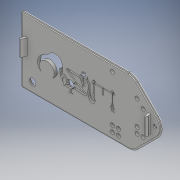
# Autodesk Inventor part: Arduino simple 4 channel ttl top
Saved by Autodesk Inventor 2017 (Build 210142000, 142)
## iProperties
Created: 2016-10-04
Part Number: Arduino simple 4 channel ttl top
Material: Generic
Document SubType Name: Modeling
Designer: andrew
Density: 1 g/cm^3
Appearance: Default
Author: andrew
Autodesk Inventor part; units mm, degrees
ref_plane "YZ Plane" through (0, 0, 0) normal (1, 0, 0) x (0, 1, 0)
ref_plane "XZ Plane" through (0, 0, 0) normal (0, 1, 0) x (-1, 0, 0)
ref_plane "XY Plane" through (0, 0, 0) normal (0, 0, 1) x (1, 0, 0)
sketch "Sketch1" plane through (0, 0, 0) normal (0, 1, 0) x (-1, 0, 0)
  line L0 (70.1002, -51.1999) -> (70.1002, -37.9894) construction
  line L1 (70.1002, -37.9894) -> (68.1002, -37.9894) construction
  line L2 (68.1002, -37.9894) -> (68.1002, -48.1999) construction
  arc A0 (67.1002, -49.1999) -> (68.1002, -48.1999) centre (67.1002, -48.1999) ccw construction
  line L3 (67.1002, -49.1999) -> (-5.9213, -49.1999) construction
  arc A1 (-7.3356, -48.6141) -> (-5.9213, -49.1999) centre (-5.9213, -47.1999) ccw construction
  line L4 (-7.3356, -48.6141) -> (-7.664, -48.2857) construction
  arc A2 (-7.664, -48.2857) -> (-9.0782, -47.6999) centre (-9.0782, -49.6999) ccw construction
  line L5 (-9.0782, -47.6999) -> (-35.9958, -47.6999) construction
  arc A3 (-42.0062, -45.2103) -> (-35.9958, -47.6999) centre (-35.9958, -39.1999) ccw construction
  line L6 (-42.0062, -45.2103) -> (-62.1562, -25.0603) construction
  arc A4 (-62.1562, -13.0395) -> (-62.1562, -25.0603) centre (-56.1458, -19.0499) ccw construction
  line L7 (-62.1562, -13.0395) -> (-42.0062, 7.1105) construction
  arc A5 (-35.9958, 9.6001) -> (-42.0062, 7.1105) centre (-35.9958, 1.1001) ccw construction
  line L8 (-35.9958, 9.6001) -> (-9.0782, 9.6001) construction
  arc A6 (-9.0782, 9.6001) -> (-7.664, 10.1859) centre (-9.0782, 11.6001) ccw construction
  line L9 (-7.664, 10.1859) -> (-7.3356, 10.5143) construction
  arc A7 (-5.9213, 11.1001) -> (-7.3356, 10.5143) centre (-5.9213, 9.1001) ccw construction
  line L10 (-5.9213, 11.1001) -> (67.1002, 11.1001) construction
  arc A8 (68.1002, 10.1001) -> (67.1002, 11.1001) centre (67.1002, 10.1001) ccw construction
  line L11 (68.1002, 10.1001) -> (68.1002, 5.7045) construction
  line L12 (68.1002, 5.7045) -> (70.1002, 5.7045) construction
  line L13 (70.1002, 5.7045) -> (70.1002, 13.1001) construction
  line L14 (70.1002, 13.1001) -> (-35.9958, 13.1001) construction
  arc A9 (-35.9958, 13.1001) -> (-44.4811, 9.5854) centre (-35.9958, 1.1001) ccw construction
  line L15 (-44.4811, 9.5854) -> (-64.6311, -10.5646) construction
  arc A10 (-64.6311, -10.5646) -> (-64.6311, -27.5352) centre (-56.1458, -19.0499) ccw construction
  line L16 (-64.6311, -27.5352) -> (-44.4811, -47.6852) construction
  arc A11 (-44.4811, -47.6852) -> (-35.9958, -51.1999) centre (-35.9958, -39.1999) ccw construction
  line L17 (-35.9958, -51.1999) -> (70.1002, -51.1999) construction
  line L18 (70.1002, -21.9894) -> (70.1002, -6.0043) construction
  line L19 (70.1002, -6.0043) -> (68.1002, -6.0043) construction
  line L20 (68.1002, -6.0043) -> (68.1002, -21.9894) construction
  line L21 (68.1002, -21.9894) -> (70.1002, -21.9894) construction
  line L22 (71.1002, -21.9894) -> (71.1002, -6.0043) construction
  line L23 (71.1002, 5.7045) -> (71.1002, 13.1001)
  arc A12 (71.1002, 13.1001) -> (70.1002, 14.1001) centre (70.1002, 13.1001) ccw
  line L24 (70.1002, 14.1001) -> (-35.9958, 14.1001)
  arc A13 (-35.9958, 14.1001) -> (-45.1882, 10.2925) centre (-35.9958, 1.1001) ccw
  line L25 (-45.1882, 10.2925) -> (-65.3382, -9.8575)
  arc A14 (-65.3382, -9.8575) -> (-65.3382, -28.2423) centre (-56.1458, -19.0499) ccw
  line L26 (-65.3382, -28.2423) -> (-45.1882, -48.3923)
  arc A15 (-45.1882, -48.3923) -> (-35.9958, -52.1999) centre (-35.9958, -39.1999) ccw
  line L27 (-35.9958, -52.1999) -> (70.1002, -52.1999)
  arc A16 (70.1002, -52.1999) -> (71.1002, -51.1999) centre (70.1002, -51.1999) ccw
  line L28 (71.1002, -51.1999) -> (71.1002, -37.9894)
  line L29 (71.1002, -37.9894) -> (70.1002, -37.9894) construction
  line L30 (70.1002, -37.9894) -> (70.1002, -51.1999) construction
  line L31 (70.1002, -51.1999) -> (-35.9958, -51.1999) construction
  arc A17 (-44.4811, -47.6852) -> (-35.9958, -51.1999) centre (-35.9958, -39.1999) ccw construction
  line L32 (-44.4811, -47.6852) -> (-64.6311, -27.5352) construction
  arc A18 (-64.6311, -10.5646) -> (-64.6311, -27.5352) centre (-56.1458, -19.0499) ccw construction
  line L33 (-64.6311, -10.5646) -> (-44.4811, 9.5854) construction
  arc A19 (-35.9958, 13.1001) -> (-44.4811, 9.5854) centre (-35.9958, 1.1001) ccw construction
  line L34 (-35.9958, 13.1001) -> (70.1002, 13.1001) construction
  line L35 (70.1002, 13.1001) -> (70.1002, 5.7045) construction
  line L36 (70.1002, 5.7045) -> (71.1002, 5.7045) construction
  line L37 (71.1002, 5.7045) -> (71.1002, 13.1001)
  line L38 (71.1002, 5.7045) -> (71.1002, -37.9894)
  arc A20 (-62.1562, -13.0395) -> (-62.1562, -25.0603) centre (-56.1458, -19.0499) ccw construction
  line L39 (-64.6458, -19.0499) -> (-76.6779, -19.0499) construction
  arc A21 (-65.3382, -9.8575) -> (-65.3382, -28.2423) centre (-56.1458, -19.0499) ccw
  circle A22 centre (-63.0458, -19.0499) radius 1.8
  point P0 (0, 0)
  point P1 (66.1, 7.6)
  point P2 (-59.329, -19.0499)
  constraints: 80 end point, 45 point on circle, 23 centre point, 1 vertical
extrude "Extrusion1" add sketch "Sketch1" along normal blind 3
sketch "Sketch2" plane through (0, 0, 0) normal (0, -1, 0) x (1, 0, 0)
  arc A0 (-71.1002, -51.1999) -> (-70.1002, -52.1999) centre (-70.1002, -51.1999) ccw projected
  line L0 (-71.1002, 13.1001) -> (-71.1002, -0.1104)
  line L1 (-70.1002, -0.1104) -> (-68.1002, -0.1104) construction
  line L2 (-68.1002, -0.1104) -> (-68.1002, 10.1001) construction
  arc A1 (-67.1002, 11.1001) -> (-68.1002, 10.1001) centre (-67.1002, 10.1001) ccw construction
  line L3 (-68.1002, -16.1104) -> (-70.1002, -16.1104) construction
  line L4 (-70.1002, -16.1104) -> (-70.1002, -32.0955) construction
  line L5 (-71.1002, -16.1104) -> (-71.1002, -32.0955) construction
  line L6 (-70.1002, -32.0955) -> (-68.1002, -32.0955) construction
  line L7 (-68.1002, -32.0955) -> (-68.1002, -16.1104) construction
  line L8 (-71.1002, -43.8043) -> (-71.1002, -0.1104)
  line L9 (-67.1002, 11.1001) -> (5.9213, 11.1001) construction
  line L10 (35.9958, 14.1001) -> (-70.1002, 14.1001)
  line L11 (35.9958, 13.1001) -> (-70.1002, 13.1001) construction
  line L12 (5.9213, -49.1999) -> (-67.1002, -49.1999) construction
  line L13 (-70.1002, -51.1999) -> (35.9958, -51.1999) construction
  line L14 (-70.1002, -52.1999) -> (35.9958, -52.1999)
  line L15 (-70.1002, 13.1001) -> (-70.1002, -0.1104) construction
  arc A2 (-70.1002, 14.1001) -> (-71.1002, 13.1001) centre (-70.1002, 13.1001) ccw
  line L16 (-68.1002, -43.8043) -> (-70.1002, -43.8043) construction
  line L17 (-68.1002, -48.1999) -> (-68.1002, -43.8043) construction
  arc A3 (-68.1002, -48.1999) -> (-67.1002, -49.1999) centre (-67.1002, -48.1999) ccw construction
  line L18 (-71.1002, -43.8043) -> (-71.1002, -51.1999)
  line L19 (-71.1002, -43.8043) -> (-71.1002, -51.1999)
  line L20 (-70.1002, -43.8043) -> (-70.1002, -51.1999) construction
  arc A4 (-71.1002, -51.1999) -> (-70.1002, -52.1999) centre (-70.1002, -51.1999) ccw
  arc A5 (5.9213, -49.1999) -> (7.3356, -48.6141) centre (5.9213, -47.1999) ccw construction
  arc A6 (9.0782, -47.6999) -> (7.664, -48.2857) centre (9.0782, -49.6999) ccw construction
  line L21 (35.9958, -47.6999) -> (9.0782, -47.6999) construction
  arc A7 (35.9958, -47.6999) -> (42.0062, -45.2103) centre (35.9958, -39.1999) ccw construction
  arc A8 (35.9958, -52.1999) -> (45.1882, -48.3923) centre (35.9958, -39.1999) ccw
  line L22 (7.664, -48.2857) -> (7.3356, -48.6141) construction
  line L23 (62.1562, -25.0603) -> (42.0062, -45.2103) construction
  line L24 (45.1882, -48.3923) -> (65.3382, -28.2423)
  arc A9 (62.1562, -25.0603) -> (62.1562, -13.0395) centre (56.1458, -19.0499) ccw construction
  arc A10 (65.3382, -28.2423) -> (65.3382, -9.8575) centre (56.1458, -19.0499) ccw
  arc A11 (7.3356, 10.5143) -> (5.9213, 11.1001) centre (5.9213, 9.1001) ccw construction
  arc A12 (7.664, 10.1859) -> (9.0782, 9.6001) centre (9.0782, 11.6001) ccw construction
  line L25 (9.0782, 9.6001) -> (35.9958, 9.6001) construction
  line L26 (7.3356, 10.5143) -> (7.664, 10.1859) construction
  line L27 (42.0062, 7.1105) -> (62.1562, -13.0395) construction
  line L28 (65.3382, -9.8575) -> (45.1882, 10.2925)
  arc A13 (42.0062, 7.1105) -> (35.9958, 9.6001) centre (35.9958, 1.1001) ccw construction
  arc A14 (44.4811, 9.5854) -> (35.9958, 13.1001) centre (35.9958, 1.1001) ccw construction
  arc A15 (45.1882, 10.2925) -> (35.9958, 14.1001) centre (35.9958, 1.1001) ccw
  line L29 (-69.6002, 12.6001) -> (35.9958, 12.6001)
  arc A16 (44.1275, 9.2318) -> (35.9958, 12.6001) centre (35.9958, 1.1001) ccw
  line L30 (44.1275, 9.2318) -> (64.2775, -10.9182)
  arc A17 (64.2775, -27.1816) -> (64.2775, -10.9182) centre (56.1458, -19.0499) ccw
  line L31 (64.2775, -27.1816) -> (44.1275, -47.3316)
  arc A18 (35.9958, -50.6999) -> (44.1275, -47.3316) centre (35.9958, -39.1999) ccw
  line L32 (35.9958, -50.6999) -> (-69.6002, -50.6999)
  line L33 (-69.6002, -50.6999) -> (-69.6002, 12.6001)
  point P0 (0, -38.0998)
  point P1 (-66.1, -45.6998)
  constraints: 68 end point, 36 point on circle, 18 centre point, 1 vertical
extrude "Extrusion2" cut sketch "Sketch2" against normal blind 1
fillet "Fillet1" radius 2 10 edges at (40.9707, 3, 13.1105) (55.2632, 3, 0.2175) (69.1458, 3, -19.0499) (55.2632, 3, -38.3173) (40.9707, 3, -51.2103) (-17.0522, 3, -52.1999) (-70.8073, 3, -51.907) (-71.1002, 3, -19.0499) (-70.8073, 3, 13.8072) (-17.0522, 3, 14.1001)
sketch "Sketch3" plane through (0, 0, 0) normal (0, -1, 0) x (1, 0, 0)
  arc A0 (65.3382, -28.2423) -> (65.3382, -9.8575) centre (56.1458, -19.0499) ccw construction
  line L0 (-70.1002, -43.8043) -> (-71.1002, -43.8043) construction
  line L1 (-70.1002, -43.8043) -> (-70.1002, -51.1999) construction
  line L2 (-70.1002, -51.1999) -> (-70.1002, -43.8043) construction
  line L3 (-68.1002, -48.1999) -> (-68.1002, -43.8043) construction
  line L4 (-68.1002, -43.8043) -> (-70.1002, -43.8043) construction
  line L5 (-70.1002, -32.0955) -> (-68.1002, -32.0955) construction
  line L6 (-71.1002, -16.1104) -> (-71.1002, -32.0955) construction
  line L7 (-70.1002, -16.1104) -> (-70.1002, -32.0955) construction
  line L8 (-68.1002, -32.0955) -> (-68.1002, -16.1104) construction
  line L9 (-68.1002, -16.1104) -> (-70.1002, -16.1104) construction
  line L10 (-71.1002, -43.8043) -> (-71.1002, -0.1104) construction
  line L11 (-70.1002, -0.1104) -> (-68.1002, -0.1104) construction
  line L12 (-68.1002, -0.1104) -> (-68.1002, 10.1001) construction
  line L13 (-70.1002, -0.1104) -> (-70.1002, 13.1001) construction
  line L14 (5.9213, -49.1999) -> (-67.1002, -49.1999) construction
  line L15 (-70.1002, -52.1999) -> (35.9958, -52.1999) construction
  line L16 (35.9958, -51.1999) -> (-70.1002, -51.1999) construction
  line L17 (-70.1002, -51.1999) -> (35.9958, -51.1999) construction
  line L18 (-67.1002, 11.1001) -> (5.9213, 11.1001) construction
  line L19 (35.9958, 13.1001) -> (-70.1002, 13.1001) construction
  line L20 (-70.1002, 13.1001) -> (35.9958, 13.1001) construction
  line L21 (35.9958, 14.1001) -> (-70.1002, 14.1001) construction
  line L22 (-71.1002, -43.8043) -> (-71.1002, -51.1999) construction
  line L23 (-71.1002, -43.8043) -> (-71.1002, -51.1999) construction
  arc A1 (-71.1002, -51.1999) -> (-70.1002, -52.1999) centre (-70.1002, -51.1999) ccw construction
  arc A2 (-68.1002, -48.1999) -> (-67.1002, -49.1999) centre (-67.1002, -48.1999) ccw construction
  arc A3 (-67.1002, 11.1001) -> (-68.1002, 10.1001) centre (-67.1002, 10.1001) ccw construction
  line L24 (-71.1002, 13.1001) -> (-71.1002, -0.1104) construction
  line L25 (-71.1002, -0.1104) -> (-70.1002, -0.1104) construction
  arc A4 (-70.1002, 14.1001) -> (-71.1002, 13.1001) centre (-70.1002, 13.1001) ccw construction
  line L26 (-70.1002, 13.1001) -> (-70.1002, -0.1104) construction
  line L27 (7.664, -48.2857) -> (7.3356, -48.6141) construction
  arc A5 (9.0782, -47.6999) -> (7.664, -48.2857) centre (9.0782, -49.6999) ccw construction
  line L28 (7.3356, 10.5143) -> (7.664, 10.1859) construction
  arc A6 (7.3356, 10.5143) -> (5.9213, 11.1001) centre (5.9213, 9.1001) ccw construction
  line L29 (35.9958, -47.6999) -> (9.0782, -47.6999) construction
  line L30 (9.0782, 9.6001) -> (35.9958, 9.6001) construction
  arc A7 (5.9213, -49.1999) -> (7.3356, -48.6141) centre (5.9213, -47.1999) ccw construction
  arc A8 (7.664, 10.1859) -> (9.0782, 9.6001) centre (9.0782, 11.6001) ccw construction
  arc A9 (64.6311, -27.5352) -> (64.6311, -10.5646) centre (56.1458, -19.0499) ccw construction
  arc A10 (35.9958, -47.6999) -> (42.0062, -45.2103) centre (35.9958, -39.1999) ccw construction
  arc A11 (35.9958, -51.1999) -> (44.4811, -47.6852) centre (35.9958, -39.1999) ccw construction
  arc A12 (35.9958, -51.1999) -> (44.4811, -47.6852) centre (35.9958, -39.1999) ccw construction
  arc A13 (35.9958, -52.1999) -> (45.1882, -48.3923) centre (35.9958, -39.1999) ccw construction
  line L31 (45.1882, -48.3923) -> (65.3382, -28.2423) construction
  line L32 (64.6311, -27.5352) -> (44.4811, -47.6852) construction
  line L33 (44.4811, -47.6852) -> (64.6311, -27.5352) construction
  arc A14 (62.1562, -25.0603) -> (62.1562, -13.0395) centre (56.1458, -19.0499) ccw construction
  arc A15 (64.6311, -27.5352) -> (64.6311, -10.5646) centre (56.1458, -19.0499) ccw construction
  arc A16 (65.3382, -28.2423) -> (65.3382, -9.8575) centre (56.1458, -19.0499) ccw construction
  line L34 (62.1562, -25.0603) -> (42.0062, -45.2103) construction
  arc A17 (42.0062, 7.1105) -> (35.9958, 9.6001) centre (35.9958, 1.1001) ccw construction
  arc A18 (44.4811, 9.5854) -> (35.9958, 13.1001) centre (35.9958, 1.1001) ccw construction
  arc A19 (44.4811, 9.5854) -> (35.9958, 13.1001) centre (35.9958, 1.1001) ccw construction
  arc A20 (45.1882, 10.2925) -> (35.9958, 14.1001) centre (35.9958, 1.1001) ccw construction
  line L35 (42.0062, 7.1105) -> (62.1562, -13.0395) construction
  line L36 (64.6311, -10.5646) -> (44.4811, 9.5854) construction
  line L37 (44.4811, 9.5854) -> (64.6311, -10.5646) construction
  line L38 (65.3382, -9.8575) -> (45.1882, 10.2925) construction
  line L39 (60.2707, -28.8292) -> (65.5374, -23.5625) construction
  circle A21 centre (63.0458, -19.0499) radius 1.6 construction
  line L40 (65.5374, -23.5625) -> (65.5374, -14.3659) construction
  arc A22 (65.3382, -28.2423) -> (65.3382, -9.8575) centre (56.1458, -19.0499) ccw construction
  line L41 (59.329, -27.8875) -> (60.2707, -28.8292) construction
  arc A23 (62.1562, -25.0603) -> (62.1562, -13.0395) centre (56.1458, -19.0499) ccw construction
  line L42 (59.329, -27.8875) -> (59.329, -10.2123) construction
  line L43 (65.5374, -14.3659) -> (59.329, -8.1575) construction
  line L44 (59.329, -8.1575) -> (59.329, -10.2123) construction
  line L45 (59.329, -19.0499) -> (80.366, -19.0499) construction
  line L46 (64.6458, -19.0499) -> (76.6779, -19.0499) construction
  line L47 (84.5257, -29.0109) -> (86.6689, -29.0109) construction
  line L48 (-67.7002, -6.1514) -> (-67.7002, -21.9095)
  line L49 (-67.7002, -21.9095) -> (-67.7002, -6.1514)
  line L50 (59.329, -27.8875) -> (58.929, -27.8875) construction
  line L51 (58.929, -27.8875) -> (58.929, -27.4875) construction
  line L52 (58.929, -27.4875) -> (56.929, -27.4875) construction
  line L53 (59.329, -10.2123) -> (58.929, -10.2123) construction
  line L54 (58.929, -10.2123) -> (58.929, -10.6123) construction
  line L55 (58.929, -27.4875) -> (58.929, -10.6123)
  line L56 (57.929, -27.4875) -> (57.929, -10.6123)
  line L57 (57.929, -27.4875) -> (58.929, -27.4875)
  line L58 (58.929, -10.6123) -> (57.929, -10.6123)
  line L59 (-66.7002, -6.1514) -> (-66.7002, -21.9095)
  line L60 (-66.7002, -21.9095) -> (-67.7002, -21.9095)
  line L61 (-66.7002, -6.1514) -> (-67.7002, -6.1514)
  line L62 (-70.1002, 14.1001) -> (35.9958, 14.1001) construction
  line L63 (-67.2002, 14.1001) -> (-67.2002, -6.0039) construction
  line L64 (-67.2002, 14.1001) -> (-47.0962, 14.1001) construction
  line L65 (-67.2002, 14.1001) -> (-67.2002, -21.9899) construction
  point P0 (-66.1, -45.6998)
  point P1 (0, -38.0998)
  dimension "d10" = 3.2
  dimension "d13" = 0.4
  dimension "d14" = 0.4
  dimension "d15" = 2
  dimension "d16" = 0.4
  dimension "d50" = 20.104
  dimension "d51" = 90
  dimension "d52" = 36.09
  constraints: 130 end point, 45 point on circle, 23 centre point, 7 perpendicular, 4 horizontal, 4 point on line, 3 parallel, 2 vertical, 1 collinear, 1 midpoint
  measures "d10" diameter of A21
  measures "d13" distance of L41.start L50.end
  measures "d14" distance of L50.end L51.end
  measures "d15" distance of L51.end L52.end
  measures "d16" distance of L53.end L54.end
  measures "d50" distance of L63.start L63.end
  measures "d51" angle of L63 L64
  measures "d52" distance of L63.start L65.end
extrude "Extrusion3" add sketch "Sketch3" along normal blind 5
sketch "Sketch7" plane through (-66.7002, 0, -21.9095) normal (0, 0, -1) x (-1, 0, 0)
  line L0 (1, 0) -> (1, -5) construction
  line L1 (1, -5) -> (1.4, -5) construction
  line L2 (1.4, -5) -> (1.9, -5) construction
  line L3 (1.9, -5) -> (1.9, -3) construction
  line L4 (1.9, -3) -> (1, -3) construction
  line L5 (1.9, -3) -> (1.9, -3.5) construction
  line L6 (1.9, -3.5) -> (0.5, -5) construction
  line L7 (0, -5) -> (1, -5) construction
  line L8 (1, -3) -> (1.9, -3)
  line L9 (1.9, -3.5) -> (1.9, -3)
  line L10 (1.9, -3.5) -> (0.5, -5)
  line L11 (0.5, -5) -> (0.5, -3)
  line L12 (0.5, -3) -> (1, -3)
  point P0 (-66.7002, 0)
  dimension "d29" = 0.4
  dimension "d30" = 0.5
  dimension "d31" = 180
  dimension "d32" = 2
  dimension "d33" = 0.5
  constraints: 22 end point, 3 collinear, 3 horizontal, 3 point on line, 1 midpoint, 1 parallel, 1 perpendicular, 1 vertical
  measures "d29" distance of L0.end L1.end
  measures "d30" distance of L1.end L2.end
  measures "d31" angle of L2 L1
  measures "d32" distance of L2.end L3.end
  measures "d33" distance of L3.end L5.end
extrude "Extrusion7" add sketch "Sketch7" against normal blind 15.758
sketch "Sketch8" plane through (-66.7002, 0, -21.9095) normal (0, 0, -1) x (-1, 0, 0)
  line L0 (1.9, -3.5) -> (1, -4.4643) projected
  line L1 (1.45, -3.9821) -> (0.4365, -5.0681)
  line L2 (0.4365, -5.0681) -> (1.45, -5.0681)
  line L3 (1.45, -5.0681) -> (1.45, -3.9821)
  point P0 (-66.7002, 0)
  point P1 (0.5, -5)
  constraints: 6 end point, 1 collinear, 1 horizontal, 1 midpoint, 1 perpendicular
extrude "Extrusion8" cut sketch "Sketch8" against normal blind 16
sketch "Sketch9" plane through (58.929, 0, -27.4875) normal (0, 0, -1) x (-1, 0, 0)
  line L0 (125.6293, 0) -> (126.6293, 0)
  line L1 (126.6293, -3) -> (126.6293, 0)
  line L2 (128.5293, 0) -> (22.9333, 0) projected
  line L3 (126.6293, -3) -> (127.5293, -3)
  line L4 (127.5293, -3) -> (127.5293, -3.5)
  line L5 (127.5293, -3.5) -> (126.1293, -5)
  line L6 (125.6293, 0) -> (125.6293, -5) projected
  line L7 (125.6293, -5) -> (125.6293, 0)
  line L8 (-12.1673, -3.3543) -> (-13.1673, -3.3543)
  line L9 (-13.1673, -6.3543) -> (-13.1673, -3.3543)
  line L10 (-13.1673, -6.3543) -> (-14.0673, -6.3543)
  line L11 (-14.0673, -6.3543) -> (-14.0673, -6.8543)
  line L12 (-14.0673, -6.8543) -> (-12.6673, -8.3543)
  line L13 (-12.1673, -8.3543) -> (-12.1673, -3.3543)
  line L14 (-12.6673, -8.3543) -> (-12.1673, -8.3543)
  line L15 (0, -5) -> (1, -5) projected
  line L16 (-0.9, -3) -> (-0.9, -3.5)
  line L17 (0, -3) -> (0, 0)
  line L18 (0, -3) -> (-0.9, -3)
  line L19 (-0.9, -3.5) -> (0.5, -5)
  line L20 (1, 0) -> (0, 0)
  line L21 (1, -5) -> (1, 0)
  line L22 (0.5, -5) -> (1, -5)
  point P0 (58.929, 0)
  constraints: 40 end point, 2 horizontal, 2 perpendicular, 1 vertical
extrude "Extrusion9" add sketch "Sketch9" against normal blind 16.875 contours L19 L16 L18 L17 L20 L21 L15
sketch "Sketch10" plane through (58.929, 0, -27.4875) normal (0, 0, -1) x (-1, 0, 0)
  line L0 (0, -4.4643) -> (-0.9, -3.5) projected
  line L1 (-0.45, -3.9821) -> (1.0587, -5.5986)
  line L2 (1.0587, -5.5986) -> (-0.45, -5.5986)
  line L3 (-0.45, -5.5986) -> (-0.45, -3.9821)
  point P0 (58.929, 0)
  constraints: 6 end point, 1 collinear, 1 horizontal, 1 midpoint, 1 perpendicular
extrude "Extrusion10" cut sketch "Sketch10" against normal blind 20
sketch "Sketch11" plane through (0, 3, 0) normal (0, 1, 0) x (1, 0, 0)
  arc A0 (65.3382, 9.8575) -> (65.3382, 28.2423) centre (56.1458, 19.0499) ccw construction
  arc A1 (65.3382, 9.8575) -> (65.3382, 28.2423) centre (56.1458, 19.0499) ccw construction
  circle A2 centre (-50.8, 43.1) radius 1.6 construction
  line L0 (-50.8, 43.1) -> (-59.26, 43.1) construction
  line L1 (-59.26, 43.1) -> (-59.26, 41.7) construction
  circle A3 centre (-59.26, 41.7) radius 3.25
  dimension "d42" = 8.46
  dimension "d43" = 1.4
  dimension "d44" = 6.5
  constraints: 4 end point, 3 centre point, 2 point on circle, 1 coincident, 1 horizontal, 1 perpendicular
  measures "d42" distance of L0.start L0.end
  measures "d43" distance of L0.end L1.end
  measures "d44" diameter of A3
extrude "Extrusion11" cut sketch "Sketch11" against normal blind 10
chamfer "Chamfer1" distance 2 angle 45 2 edges at (-62.51, 3, -41.7) (64.8458, 3, -19.0499)
chamfer "Chamfer2" distance 2 distance2 5 1 edges at (-66.7002, 0, -14.0305) measured on face at (-66.2002, 0, -14.0305)
chamfer "Chamfer3" distance 2 distance2 5 1 edges at (57.929, 0, -19.0499) measured on face at (57.429, 0, -19.0499)
sketch "Sketch13" plane through (0, 3, 0) normal (0, 1, 0) x (1, 0, 0)
  circle A0 centre (-59.26, 41.7) radius 5.25 projected
  arc A1 (35.9958, -12.1001) -> (43.7739, -8.8783) centre (35.9958, -1.1001) ccw construction
  line L0 (63.9239, 11.2717) -> (43.7739, -8.8783) construction
  arc A2 (63.9239, 11.2717) -> (63.9239, 26.8281) centre (56.1458, 19.0499) ccw projected
  line L1 (43.7739, 46.9781) -> (63.9239, 26.8281) construction
  arc A3 (43.7739, 46.9781) -> (35.9958, 50.1999) centre (35.9958, 39.1999) ccw construction
  line L2 (-69.1002, 50.1999) -> (35.9958, 50.1999) construction
  line L3 (-69.1002, -12.1001) -> (-69.1002, 50.1999) projected
  line L4 (35.9958, -12.1001) -> (-69.1002, -12.1001) construction
  circle A4 centre (63.0458, 19.0499) radius 3.8 construction
  line L5 (-61.1312, -4.131) -> (-61.1312, 42.2308)
  line L6 (-61.1312, 42.2308) -> (35.9958, 42.2308) construction
  arc A5 (38.139, 41.3431) -> (35.9958, 42.2308) centre (35.9958, 39.1999) ccw construction
  line L7 (38.139, 41.3431) -> (58.289, 21.1931) construction
  arc A6 (58.289, 16.9067) -> (58.289, 21.1931) centre (56.1458, 19.0499) ccw construction
  line L8 (58.289, 16.9067) -> (38.139, -3.2433) construction
  arc A7 (35.9958, -4.131) -> (38.139, -3.2433) centre (35.9958, -1.1001) ccw construction
  line L9 (35.9958, -4.131) -> (-61.1312, -4.131) construction
  line L10 (23.5753, -4.131) -> (23.5753, 42.2308) construction
  line L11 (48.214, 6.8317) -> (48.214, 31.2681) construction
  line L12 (19.5753, 38.2308) -> (19.5753, 46.2308) construction
  line L13 (19.5753, 46.2308) -> (27.5753, 46.2308) construction
  line L14 (27.5753, 46.2308) -> (27.5753, 38.2308) construction
  line L15 (27.5753, 38.2308) -> (19.5753, 46.2308) construction
  line L16 (23.5753, 42.2308) -> (27.5753, 46.2308) construction
  circle A8 centre (20.5753, -7.131) radius 2
  circle A9 centre (45.214, 3.8317) radius 2
  circle A10 centre (51.214, 9.8317) radius 2
  circle A11 centre (45.214, 28.2681) radius 2
  circle A12 centre (45.214, 34.2681) radius 2
  circle A13 centre (51.214, 34.2681) radius 2
  circle A14 centre (20.5753, 39.2308) radius 2
  line L17 (20.5753, 39.2308) -> (20.5753, 45.2308) construction
  line L18 (20.5753, 45.2308) -> (26.5753, 45.2308) construction
  line L19 (26.5753, 45.2308) -> (26.5753, 39.2308) construction
  circle A15 centre (20.5753, 45.2308) radius 2
  circle A16 centre (26.5753, 45.2308) radius 2
  circle A17 centre (26.5753, 39.2308) radius 2
  line L20 (26.5753, 39.2308) -> (20.5753, 45.2308) construction
  line L21 (23.5753, 42.2308) -> (26.5753, 45.2308) construction
  point P0 (0, 0)
  dimension "d87" = 8
  dimension "d88" = 8
  dimension "d92" = 4
  dimension "d93" = 4
  dimension "d94" = 4
  dimension "d95" = 4
  dimension "d96" = 4
  dimension "d97" = 4
  dimension "d98" = 4
  dimension "d99" = 6
  dimension "d100" = 6
  dimension "d101" = 4
  dimension "d102" = 4
  dimension "d103" = 4
  constraints: 34 end point, 13 centre point, 7 perpendicular, 6 point on circle, 5 coincident, 4 midpoint, 4 point on line, 2 vertical, 7 other
  measures "d87" distance of L12.start L12.end
  measures "d88" distance of L12.end L14.start
  measures "d92" diameter of A8
  measures "d93" diameter of A9
  measures "d94" diameter of A10
  measures "d95" diameter of A11
  measures "d96" diameter of A12
  measures "d97" diameter of A13
  measures "d98" diameter of A14
  measures "d99" distance of L17.start L17.end
  measures "d100" distance of L17.end L19.start
  measures "d101" diameter of A15
  measures "d102" diameter of A16
  measures "d103" diameter of A17
extrude "Extrusion13" cut sketch "Sketch13" against normal blind 10 contours A8 | A9 | A10 | A11 | A12 | A13 | A14 | A15 | A16 | A17
sketch "Sketch16" plane through (0, 3, 0) normal (0, 1, 0) x (1, 0, 0)
  spline S0 degree 4 poles (-33.2856, 20.6534) (-34.7175, 21.9034) (-35.3641, 25.4722) (-36.932, 26.5694) (-39.0909, 28.3535) knots 0 0 0 0 0 1 1 1 1 1
  arc A0 (-51.0825, 28.3535) -> (-39.0909, 28.3535) centre (-45.0867, 23.9604) ccw
  arc A1 (-51.0825, 28.3535) -> (-49.2903, 13.197) centre (-45.0867, 21.3783) ccw
  spline S1 degree 4 poles (-49.2903, 13.197) (-48.8593, 11.9483) (-45.3246, 11.0183) (-44.582, 10.9223) (-40.7964, 6.7036) (-38.72, 5.8729) (-36.7056, 6.0529) (-34.5311, 6.3837) knots 0 0 0 0 0 0.350642 0.490165 0.626905 1 1 1 1 1
  arc A2 (-34.5311, 6.3837) -> (-30.1825, 10.2794) centre (-36.0622, 12.4678) ccw
  spline S2 degree 4 poles (-30.1825, 10.2794) (-29.5696, 13.0335) (-28.3417, 18.3439) (-30.0591, 18.3193) (-30.0692, 21.0255) (-30.2077, 21.7073) (-29.635, 21.6818) (-29.0003, 21.4179) (-28.6861, 22.2578) (-28.8113, 23.6882) (-29.4147, 24.2479) (-28.8702, 26.1714) (-29.0004, 26.6864) (-28.1892, 27.494) knots 0 0 0 0 0 0.314054 0.389387 0.450233 0.504553 0.55243 0.610485 0.672651 0.739633 0.811347 1 1 1 1 1
  spline S3 degree 3 poles (-28.1892, 27.494) (-28.9772, 27.5641) (-30.1554, 24.4132) (-29.6388, 23.3715) knots 0 0 0 0 1 1 1 1
  spline S4 degree 4 poles (-29.6388, 23.3715) (-30.1623, 22.3644) (-30.2897, 26.0625) (-34.1179, 18.8176) (-29.9101, 18.8153) (-31.1791, 16.5275) knots 0 0 0 0 0 0.383586 1 1 1 1 1
  spline S5 degree 4 poles (-31.1791, 16.5275) (-31.5178, 16.5117) (-31.3643, 15.0683) (-32.5525, 16.6963) (-32.7135, 16.3913) (-32.9963, 20.9985) (-33.2856, 20.6534) knots 0 0 0 0 0 0.307527 0.453737 1 1 1 1 1
  spline S6 degree 3 poles (-24.5536, 22.2843) (-26.2885, 23.5621) (-27.0276, 19.8418) (-28.1892, 19.8724) knots 0 0 0 0 1 1 1 1
  spline S7 degree 2 poles (-28.1892, 19.8724) (-28.83, 18.9251) (-28.1461, 19.103) knots 0 0 0 1 1 1
  spline S8 degree 3 poles (-28.1461, 19.103) (-28.0883, 19.1043) (-27.9741, 19.1145) (-27.8389, 19.1442) (-27.6856, 19.1921) (-27.5452, 19.2542) (-27.3585, 19.3637) (-27.2145, 19.4733) (-27.0539, 19.6186) (-26.938, 19.7402) (-26.7765, 19.9283) (-26.6284, 20.1227) (-26.4195, 20.42) (-26.2437, 20.6849) (-26.0308, 21.0009) (-25.8654, 21.2337) (-25.6879, 21.4546) (-25.5769, 21.5734) (-25.4774, 21.6641) (-25.4183, 21.71) (-25.3628, 21.7456) (-25.3329, 21.7609) (-25.309, 21.7711) (-25.2959, 21.7756) (-25.2827, 21.7792) (-25.2742, 21.7808) (-25.265, 21.7819) (-25.2581, 21.7822) (-25.2482, 21.7819) (-25.2387, 21.7809) (-25.2229, 21.7779) (-25.2067, 21.7736) (-25.1757, 21.7628) (-25.1219, 21.7392) (-25.0544, 21.6975) (-25.0099, 21.6647) knots 0 0 0 0 0.020676 0.041353 0.051691 0.082705 0.103382 0.144734 0.165411 0.206763 0.22744 0.289469 0.330821 0.413526 0.454879 0.537584 0.578937 0.640966 0.661642 0.702995 0.723671 0.754686 0.765024 0.7857 0.796038 0.816715 0.827053 0.847729 0.858067 0.878744 0.889082 0.909758 0.920096 0.951111 0.992463 0.992463 0.992463 0.992463
  spline S9 degree 2 poles (-25.0099, 21.6647) (-24.5127, 21.6436) (-23.8297, 21.7203) knots 0 0 0 1 1 1
  arc A3 (-23.8297, 21.7203) -> (-18.4763, 23.0471) centre (-21.8146, 25.0531) ccw
  spline S10 degree 4 poles (-18.4763, 23.0471) (-17.7175, 21.2585) (-18.6444, 22.064) (-15.4356, 19.6671) (-14.555, 23.3221) (-16.6527, 21.742) (-16.5188, 22.2357) (-17.5048, 22.3983) knots 0 0 0 0 0 0.398573 0.540898 0.679309 1 1 1 1 1
  spline S11 degree 2 poles (-17.5048, 22.3983) (-18.1667, 22.3996) (-18.0185, 24.1827) knots 0 0 0 1 1 1
  arc A4 (-18.0185, 24.1827) -> (-17.9202, 25.0951) centre (-21.8146, 25.0531) ccw
  spline S12 degree 3 poles (-17.9202, 25.0951) (-14.4576, 24.925) (-13.532, 25.2311) (-7.3325, 25.5435) knots 0 0 0 0 1 1 1 1
  line L0 (-7.3325, 25.5435) -> (-25.1614, 14.3914)
  spline S13 degree 2 poles (-25.1614, 14.3914) (-25.4523, 13.4381) (-24.5536, 12.4678) knots 0 0 0 1 1 1
  line L1 (-24.5536, 12.4678) -> (-12.9994, 12.9453)
  line L2 (-13.0592, 14.3914) -> (-23.5799, 13.9566)
  line L3 (-23.5799, 13.9566) -> (-6.003, 24.9422)
  spline S14 degree 4 poles (-6.003, 24.9422) (-5.2047, 25.5435) (-5.0509, 26.3987) (-5.6134, 27.2979) (-6.8413, 27.3893) (-9.8139, 27.2979) (-14.0046, 26.8239) (-16.0064, 26.8008) (-16.9515, 26.8392) (-17.3414, 26.9007) knots 1 1 1 1 1 2 3 4 5 6 6.802438 6.802438 6.802438 6.802438 6.802438
  spline S15 degree 4 poles (-17.3414, 26.9007) (-17.4374, 26.9158) (-18.0079, 27.0239) (-18.5299, 27.2493) (-19.1487, 27.7383) (-20.2082, 28.6009) knots 6.802438 6.802438 6.802438 6.802438 6.802438 7 8 8 8 8 8
  spline S16 degree 3 poles (-20.2082, 28.6009) (-20.5167, 29.7894) (-20.647, 31.9945) (-19.8207, 31.5984) knots 0 0 0 0 1 1 1 1
  spline S17 degree 4 poles (-19.8207, 31.5984) (-19.4499, 31.1709) (-18.4003, 31.6065) (-20.0527, 33.3292) (-20.5046, 31.3169) (-21.8834, 31.6395) (-21.7557, 32.1542) knots 0 0 0 0 0 0.393852 0.564941 1 1 1 1 1
  spline S18 degree 4 poles (-21.7557, 32.1542) (-21.3729, 32.9759) (-23.9302, 33.2582) (-22.6898, 31.1639) (-20.8, 31.1995) (-21.7679, 30.1696) (-21.2457, 29.0005) (-21.0973, 28.881) knots 0 0 0 0 0 0.379017 0.523779 0.680013 0.97265 0.97265 0.97265 0.97265 0.97265
  arc A5 (-21.0973, 28.881) -> (-23.5799, 28.5246) centre (-21.8146, 25.0531) ccw
  spline S19 degree 2 poles (-23.5799, 28.5246) (-24.5793, 28.7257) (-25.3859, 28.3491) knots 0 0 0 1 1 1
  spline S20 degree 3 poles (-25.3859, 28.3491) (-25.4311, 28.3487) (-25.5259, 28.3524) (-25.6558, 28.3687) (-25.7938, 28.3941) (-25.9101, 28.4217) (-26.0618, 28.4647) (-26.1877, 28.5056) (-26.3496, 28.5641) (-26.4822, 28.6161) (-26.6509, 28.6864) (-26.788, 28.7464) (-26.9959, 28.8402) (-27.2768, 28.9703) (-27.5277, 29.0849) (-27.6744, 29.1473) knots 0.113605 0.113605 0.113605 0.113605 0.185987 0.258369 0.29456 0.366942 0.403132 0.475514 0.511705 0.584087 0.620278 0.69266 0.72885 0.837423 0.982187 0.982187 0.982187 0.982187
  spline S21 degree 2 poles (-27.6744, 29.1473) (-28.9893, 28.8761) (-28.1467, 28.1681) knots 0 0 0 1 1 1
  spline S22 degree 3 poles (-28.1467, 28.1681) (-27.2667, 27.8011) (-26.106, 27.0999) (-24.9971, 27.2979) knots 0 0 0 0 1 1 1 1
  arc A6 (-24.9971, 27.2979) -> (-24.5536, 22.2843) centre (-21.8146, 25.0531) ccw
  line L4 (1.4817, 21.7263) -> (1.4817, 12.2341)
  line L5 (1.4817, 12.2341) -> (0.8381, 13.2226)
  line L6 (0.8381, 13.2226) -> (-0.3159, 11.8853)
  line L7 (-0.3159, 11.8853) -> (2.1964, 9.0617)
  line L8 (2.1964, 9.0617) -> (3.5871, 10.2991)
  line L9 (3.5871, 10.2991) -> (2.5828, 11.4279)
  line L10 (2.5828, 11.4279) -> (20.6352, 11.4279)
  line L11 (20.6352, 11.4279) -> (19.4088, 10.1175)
  line L12 (19.4088, 10.1175) -> (20.4913, 8.9009)
  line L13 (20.4913, 8.9009) -> (23.3314, 11.4279)
  line L14 (23.3314, 11.4279) -> (21.8942, 12.773)
  line L15 (21.8942, 12.773) -> (20.9518, 11.7661)
  line L16 (20.9518, 11.7661) -> (20.9518, 19.4716)
  line L17 (20.9518, 19.4716) -> (20.4913, 19.7316)
  line L18 (20.242, 19.8724) -> (20.1887, 12.1004)
  line L19 (20.1887, 12.1004) -> (11.609, 12.1592)
  line L20 (11.609, 12.1592) -> (11.609, 18.105)
  line L21 (11.609, 18.105) -> (10.7204, 18.2495)
  line L22 (10.7204, 18.2495) -> (10.6787, 12.1655)
  line L23 (10.6787, 12.1655) -> (2.1964, 12.2236)
  line L24 (2.1964, 12.2236) -> (2.261, 21.6659)
  spline S23 degree 4 poles (2.261, 21.6659) (2.3403, 21.6847) (2.5944, 21.7772) (2.873, 22.0723) (2.873, 22.451) (2.1857, 22.8433) (2.1857, 23.4529) (2.1857, 24.7099) (3.0514, 25.649) (3.2915, 27.2979) (2.7647, 29.2266) (1.8094, 30.0165) (-0.5849, 30.3864) (-3.7532, 27.9603) (-4.5103, 22.6606) (-3.484, 18.5854) (-2.9866, 16.5105) (-3.3126, 15.9054) (-3.5259, 15.794) (-3.6118, 15.7782) knots 5.292479 5.292479 5.292479 5.292479 5.292479 5.692476 6.692476 7.692476 8.692476 9.692476 10.692476 11.692476 12.692476 13.692476 14.692476 15.692476 16.692476 17.692476 18.692476 19.692476 20.399997 20.399997 20.399997 20.399997 20.399997
  spline S24 degree 4 poles (-3.6118, 15.7782) (-4.0479, 15.8497) (-4.5394, 15.6358) (-4.8647, 14.5298) (-4.634, 13.5788) (-4.4, 11.8559) (-4.7759, 10.8635) (-5.2047, 9.8944) knots 1 1 1 1 1 2 3 4 5 5 5 5 5
  spline S25 degree 4 poles (-5.2047, 9.8944) (-4.2478, 10.7727) (-3.7532, 12.3551) (-3.8024, 14.0045) (-3.5689, 14.3778) (-3.2661, 14.1934) knots 1 1 1 1 1 2 3 3 3 3 3
  spline S26 degree 4 poles (-3.2661, 14.1934) (-3.2347, 14.1821) (-3.0879, 14.0961) (-2.8301, 13.7093) (-2.2297, 13.2821) (-1.782, 14.8675) (-1.8982, 16.1264) (-1.8982, 19.4716) (-1.5488, 22.9256) (-0.6053, 25.8664) (0.4869, 27.0844) (1.7721, 27.6943) (2.3758, 26.7992) (2.1964, 25.5435) (1.621, 24.636) (1.3425, 23.3715) (0.8381, 22.9256) (0.2634, 22.551) (0.8288, 22.0117) (1.283, 21.792) (1.4817, 21.7263) knots 21.225328 21.225328 21.225328 21.225328 21.225328 21.495604 22.495604 23.495604 24.495604 25.495604 26.495604 27.495604 28.495604 29.495604 30.495604 31.495604 32.495604 33.495604 34.495604 35.495604 36.495604 37.270276 37.270276 37.270276 37.270276 37.270276
  spline S27 degree 4 poles (-12.9994, 12.9453) (-12.2362, 12.4678) (-10.878, 10.7969) (-9.8742, 10.4388) (-10.1104, 8.7855) (-8.9785, 6.9759) (-7.9975, 7.5896) (-8.6342, 9.0217) (-8.6342, 10.0238) (-7.5122, 9.3169) (-6.7123, 8.038) (-7.5713, 6.5255) (-5.9154, 8.3721) (-5.9154, 9.4382) (-7.3325, 10.7969) (-7.9256, 11.2655) (-8.6342, 11.6508) (-6.6935, 11.6508) (-5.3114, 12.4678) (-5.9154, 13.8046) (-6.6124, 13.4732) (-6.6124, 12.9453) (-7.7484, 12.4678) (-8.6932, 12.9453) (-9.1162, 13.6215) (-8.1027, 14.8675) (-6.2785, 14.8675) (-5.62, 15.9418) (-6.9808, 16.1666) (-8.6932, 15.458) (-8.6932, 16.7949) (-6.8954, 17.9194) (-5.9154, 18.487) (-6.6817, 19.5691) (-7.9639, 18.7421) (-8.6932, 17.9381) (-8.1618, 20.6503) (-9.4583, 21.7203) (-9.6971, 20.6503) (-9.4583, 19.2158) (-10.1694, 18.4695) (-11.1142, 17.1704) (-10.878, 15.8967) (-11.8819, 13.4732) (-13.0592, 14.3914) knots 1 1 1 1 1 2 3 4 5 6 7 8 9 10 11 12 13 14 15 16 17 18 19 20 21 22 23 24 25 26 27 28 29 30 31 32 33 34 35 36 37 38 39 40 41 42 42 42 42 42
  line L25 (20.4913, 19.7316) -> (21.7569, 21.7263)
  line L26 (21.7569, 21.7263) -> (20.4913, 21.7263)
  line L27 (20.4913, 21.7263) -> (22.6128, 24.7099)
  line L28 (22.6128, 24.7099) -> (20.8358, 24.7099)
  line L29 (20.8358, 24.7099) -> (22.6128, 27.2089)
  line L30 (22.6128, 27.2089) -> (19.9671, 27.2089)
  line L31 (19.9671, 27.2089) -> (18.6476, 23.699)
  line L32 (18.6476, 23.699) -> (19.9671, 23.699)
  line L33 (19.9671, 23.699) -> (19.1256, 21.4607)
  line L34 (19.1256, 21.4607) -> (20.4913, 21.1305)
  line L35 (20.4913, 21.1305) -> (20.242, 19.8724)
  point P0 (0, 0)
  constraints: 72 end point, 14 point on circle, 7 centre point, 77 other
extrude "Extrusion15" cut sketch "Sketch16" against normal blind 10
body "Solid1"
